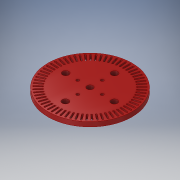
# Autodesk Inventor part: Деталь1
Saved by Autodesk Inventor 2019 (Build 230136000, 136)
## iProperties
Created: 2019-05-20
Part Number: Деталь1
Material: Пластик АБС
Document SubType Name: Modeling
Designer: User
Density: 1.06 g/cm^3
Appearance: Красный
Author: User
Autodesk Inventor part; units mm, degrees
ref_plane "YZ Plane" through (0, 0, 0) normal (1, 0, 0) x (0, 1, 0)
ref_plane "XZ Plane" through (0, 0, 0) normal (0, 1, 0) x (-1, 0, 0)
ref_plane "XY Plane" through (0, 0, 0) normal (0, 0, 1) x (1, 0, 0)
sketch "Эскиз1" plane through (0, 0, 0) normal (0, 1, 0) x (-1, 0, 0)
  circle A0 centre (0, 0) radius 27.5
  dimension "d0" = 55
  constraints: 1 centre point, 1 coincident
  measures "d0" diameter of A0
extrude "Выдавливание1" add sketch "Эскиз1" along normal blind 3
sketch "Эскиз2" plane through (0, 3, 0) normal (0, 1, 0) x (1, 0, 0)
  circle A0 centre (0, 0) radius 2
  line L0 (0, 0) -> (0, -8)
  circle A1 centre (0, -8) radius 1
  circle A2 centre (8, 0) radius 1
  circle A3 centre (0, 8) radius 1
  circle A4 centre (-8, 0) radius 1
  dimension "d3" = 4
  dimension "d4" = 8
  dimension "d5" = 2
  dimension "d8" = 360
  constraints: 5 centre point, 2 coincident, 2 end point, 1 vertical, 9 other
  measures "d3" diameter of A0
  measures "d4" distance of L0.start L0.end
  measures "d5" diameter of A1
extrude "Выдавливание2" cut sketch "Эскиз2" against normal blind 4
sketch "Эскиз5" plane through (0, 3, 0) normal (0, 1, 0) x (1, 0, 0)
  line L0 (0, 0) -> (0, 10)
  line L1 (0, 10) -> (-1.5, 10)
  circle A0 centre (0, 0) radius 10
  line L2 (-1.5107, 18.736) -> (1.4893, 18.736) construction
  line L3 (-1.5, 10) -> (1.4893, 10)
  line L4 (1.4893, 18.736) -> (-1.5, 18.736)
  line L5 (-1.5, 18.736) -> (-1.5, 10)
  line L6 (1.4893, 10) -> (1.4893, 18.736)
  line L7 (0.0054, 26.132) -> (-0.0054, 21.868) construction
  line L8 (-0.4946, 26.1333) -> (-0.5054, 21.8693)
  line L9 (0.4946, 21.8667) -> (0.5054, 26.1307)
  arc A1 (0.5054, 26.1307) -> (-0.4946, 26.1333) centre (0.0054, 26.132) ccw
  arc A2 (-0.5054, 21.8693) -> (0.4946, 21.8667) centre (-0.0054, 21.868) ccw
  line L10 (-1.5, 18.736) -> (1.4893, 10)
  line L11 (-1.5331, 9.8818) -> (1.4893, 18.736)
  point P0 (-1, 10)
  point P1 (0, 9.8794)
  point P2 (1.467, 9.8918)
  point P3 (0, 24)
  dimension "d23" = 1.5
  dimension "d24" = 0.5
  dimension "d27" = 20
  dimension "d39" = 1
  dimension "d40" = 10
  dimension "d41" = 24
  constraints: 26 end point, 6 point on circle, 4 tangent, 3 centre point, 3 point on line, 2 horizontal, 2 parallel, 2 vertical, 1 coincident, 1 midpoint, 1 perpendicular
  measures "d23" distance of L0.end L1.end
  measures "d24" distance of L1.end point (-1, 10)
  measures "d27" diameter of A0
  measures "d39" distance between parallel lines of L9 L8
  measures "d40" distance of L0.start L0.end
  measures "d41" distance of L0.start point (0, 24)
extrude "Выдавливание4" cut sketch "Эскиз5" against normal blind 10 contours A1 L9 A2 L8
pattern_circular "Круговой массив3" count 65 over 360 about axis through (0, 3, 0) along (0, -1, 0) of "Выдавливание4"
sketch "Эскиз6" plane through (0, 3, 0) normal (0, 1, 0) x (1, 0, 0)
  arc A0 (-14.8717, -1.6857) -> (-18.0997, 0.0968) centre (-15.9998, 0.0856) ccw
  arc A1 (-6.8718, -1.7285) -> (-9.1468, -1.7163) centre (-7.9999, 0.0428) ccw
  circle A2 centre (0, 0) radius 4
  arc A3 (-1.7285, 6.8718) -> (-1.7163, 9.1468) centre (0.0428, 7.9999) ccw
  arc A4 (-1.6857, 14.8717) -> (0.0968, 18.0997) centre (0.0856, 15.9998) ccw
  arc A5 (6.8718, 1.7285) -> (9.1468, 1.7163) centre (7.9999, -0.0428) ccw
  arc A6 (14.8717, 1.6857) -> (18.0997, -0.0968) centre (15.9998, -0.0856) ccw
  arc A7 (1.7285, -6.8718) -> (1.7163, -9.1468) centre (-0.0428, -7.9999) ccw
  arc A8 (1.6857, -14.8717) -> (-0.0968, -18.0997) centre (-0.0856, -15.9998) ccw
  circle A9 centre (-15.9998, 0.0856) radius 2.1
  circle A10 centre (-7.9999, 0.0428) radius 2.1
  circle A11 centre (0, 0) radius 4
  circle A12 centre (0.0428, 7.9999) radius 2.1
  circle A13 centre (0.0856, 15.9998) radius 2.1
  circle A14 centre (7.9999, -0.0428) radius 2.1
  circle A15 centre (15.9998, -0.0856) radius 2.1
  circle A16 centre (-0.0428, -7.9999) radius 2.1
  circle A17 centre (-0.0856, -15.9998) radius 2.1
  dimension "d42" = 4.2
  constraints: 18 centre point, 16 point on circle, 9 coincident, 4 concentric
  measures "d42" diameter of A14
extrude "Выдавливание5" cut sketch "Эскиз6" against normal blind 10 contours A9 A0 | A13 A4 | A15 A6 | A17 A8
